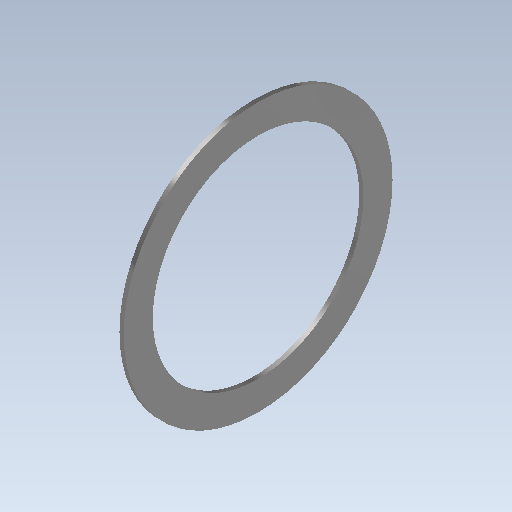
# Autodesk Inventor part: MF85ZZ Shield2
Saved by Autodesk Inventor 2020 (Build 240168000, 168)
## iProperties
Created: 2016-04-26
Part Number: MF85ZZ Shield2
Catalog Web Link: www.cadenas.de
Description: shielded_type_zz_zzs_S2-
Vendor: NSK_RB
Document SubType Name: Modeling
Designer: psAdmin
Manufacturer: NSK_RB
Mass: 0.0150569 g
Surface Area: 0.380323 cm^2
Volume: 0.00194282 cm^3
Density: 7.75 g/cm^3
Material: ステンレス鋼 440C
Appearance: 半つや出し
Category: PARTsolutions
Company: NSK_RB
PSOL_IDENT_0: {$CADENAS_DATA\23d-libs\nsk_rb\roller_bearings\deep_groove_bb\exstra_small_miniatur_bb\metric_design
PSOL_IDENT_1: _with_flange\shielded_type_zz_zzs_s2_1.prj},188 {VTYP=3D},{NB=MF85ZZ Shield2},{LINA=MF85ZZ Shield2},
PSOL_IDENT_2: {NN=shielded_type_zz_zzs_S2},{DATE=18.06.2013 02:54:38},{GEOMDATE=04.01.2008 00:00:00},{VERSION=},{L
PSOL_IDENT_3: INEID=210},{LINESUBID=-1},{WBVAR=}  {NB=MF85ZZ Shield2},{LINA=MF85ZZ Shield2},{KT=DUMMY},{IDNR=},{ST
PSOL_IDENT_4: AN=},{ORDER=MF85ZZ},{SD=5.0},{X=5.0},{D=8},{DD=8},{DD1=0.0},{D2=9.2},{DD2=9.2},{B=0.0},{B1=2.5},{CC1=
PSOL_IDENT_5: 0.0},{C2=0.6},{CC2=0.6},{R=0.00},{R1=0.10},{DI1=5.80},{DI2=5.80},{SDE1=7.00},{SDE2=7.40},{CR1=310},{
PSOL_IDENT_6: COR1=120},{CR2=31},{COR2=12.0},{LG=53000},{LO=63000},{DA=0.0},{DB=5.8},{RA=0.00},{RB=0.10},{MASS=0.4
PSOL_IDENT_7: 1},{SC=1}
NN: shielded_type_zz_zzs_S2
NB: MF85ZZ Shield2
NBSYN: $ORDER. Shield2
LINA: MF85ZZ Shield2
ORDER: MF85ZZ
SD: 5.0
X: 5.0
D: 8
DD: 8
DD1: 0.0
D2: 9.2
DD2: 9.2
B: 0.0
B1: 2.5
CC1: 0.0
C2: 0.6
CC2: 0.6
R: 0.00
R1: 0.10
DI1: 5.80
DI2: 5.80
SDE1: 7.00
SDE2: 7.40
CR1: 310
COR1: 120
CR2: 31
COR2: 12.0
LG: 53000
LO: 63000
DA: 0.0
DB: 5.8
RA: 0.00
RB: 0.10
MASS: 0.41
SC: 1
SUPPLIER: NSK_RB
ARTICLENO: MF85ZZ Shield2
BOMINFO: MF85ZZ Shield2
CREATOR: CADENAS GmbH
Title: MF85ZZ Shield2
Author: Cadenas PARTsolutions
Autodesk Inventor part; units mm, degrees
sketch "Sketch_1" plane through (0, 0, 0) normal (0, 0, 1) x (1, 0, 0)
  line L0 (2.4609, 0) -> (2.3438, 0)
  line L1 (2.3438, 2.9) -> (2.4609, 2.9)
  line L2 (2.4609, 2.9) -> (2.4609, 3.7)
  line L3 (2.4609, 3.7) -> (2.3438, 3.7)
  line L4 (2.3438, 3.7) -> (2.3438, 2.9)
  constraints: 10 end point
revolve "Revolution1" add sketch "Sketch_1" angle 360 about axis through (2.4609, 0, 0) along (1, 0, 0)
ref_plane "ip_st_1_XY" through (2.3438, 0, 0) normal (1, 0, 0) x (0, 0, -1)
ref_plane "ip_st_1_YZ" through (2.3438, 0, 0) normal (0, 0, -1) x (0, 1, 0)
ref_plane "ip_st_1_ZX" through (2.3438, 0, 0) normal (0, 1, 0) x (1, 0, 0)
body "Solid1"
